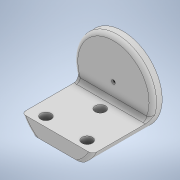
# Autodesk Inventor part: Adapter_Handgelenk
Saved by Autodesk Inventor 2022.2 (Build 262287010, 287A)
## iProperties
Created: 2024-02-12
Part Number: Adapter_Handgelenk
Material: Generisch
Document SubType Name: Modeling
Designer: ppovolni
Density: 1 g/cm^3
Appearance: Vorgabe
Author: ppovolni
Autodesk Inventor part; units mm, degrees
ref_plane "YZ Plane" through (0, 0, 0) normal (1, 0, 0) x (0, 1, 0)
ref_plane "XZ Plane" through (0, 0, 0) normal (0, 1, 0) x (-1, 0, 0)
ref_plane "XY Plane" through (0, 0, 0) normal (0, 0, 1) x (1, 0, 0)
sketch "Skizze1" plane through (0, 0, 0) normal (0, 0, 1) x (1, 0, 0)
  circle A0 centre (0, 0) radius 21
  dimension "d0" = 42
  constraints: 1 centre point, 1 coincident
  measures "d0" diameter of A0
extrude "Extrusion1" add sketch "Skizze1" along normal blind 5
sketch "Skizze2" plane through (0, 0, 0) normal (0, 0, -1) x (-1, 0, 0)
  circle A0 centre (0, 0) radius 2.35
  dimension "d3" = 4.7
  constraints: 1 centre point, 1 coincident
  measures "d3" diameter of A0
extrude "Extrusion2" cut sketch "Skizze2" against normal blind 4
sketch "Skizze3" plane through (0, 0, 4) normal (0, 0, -1) x (-1, 0, 0)
  circle A0 centre (0, 0) radius 1
  dimension "d6" = 2
  constraints: 1 centre point, 1 coincident
  measures "d6" diameter of A0
extrude "Extrusion3" cut sketch "Skizze3" against normal through all
sketch "Skizze4" plane through (0, 0, 5) normal (0, 0, 1) x (1, 0, 0)
  circle A0 centre (0, 0) radius 21 projected
  line L0 (-19, -8.9443) -> (19, -8.9443)
  dimension "d10" = 38
  constraints: 2 end point, 2 point on circle, 1 horizontal
  measures "d10" distance of L0.start L0.end
extrude "Extrusion4" add sketch "Skizze4" along normal blind 30 contours L0 A0 picked at (-5.5035, -10.2886)
fillet "Rundung1" radius 2 4 edges at (0, -8.9443, 5) (20.4939, -4.5826, 5) (-4.5826, 20.4939, 5) (0, -21, 35)
sketch "Skizze5" plane through (-17.6855, -8.9443, 7) normal (0, 1, 0) x (1, 0, 0)
  line L0 (15.3355, 7) -> (20.0355, 7) construction
  line L1 (-3.3145, 7) -> (38.6855, 7) construction
  line L2 (6.6855, 7) -> (28.6855, 7) construction
  line L3 (28.6855, 7) -> (28.6855, -23) construction
  line L4 (28.6855, -23) -> (6.6855, -23) construction
  line L5 (6.6855, -23) -> (6.6855, 7) construction
  line L6 (6.6855, -5) -> (28.6855, -5) construction
  circle A0 centre (17.6855, -5) radius 2.8
  circle A1 centre (28.6855, -23) radius 2.8
  circle A2 centre (6.6855, -23) radius 2.8
  line L7 (-1.3145, 0.1936) -> (-1.3145, -26) construction
  line L8 (36.6855, 0.1936) -> (36.6855, -26) construction
  line L9 (-1.3145, -26) -> (36.6855, -26) construction
  point P0 (17.6855, 7)
  point P1 (17.6855, -5)
  point P2 (17.6855, -26)
  dimension "d14" = 22
  dimension "d18" = 5.6
  dimension "d21" = 12
  dimension "d22" = 18
  dimension "d23" = 38
  constraints: 12 end point, 3 centre point, 3 coincident, 3 point on line, 2 equal radius, 2 horizontal, 2 midpoint, 2 parallel, 2 perpendicular, 1 vertical alignment
  measures "d14" distance of L3.end L4.end
  measures "d18" diameter of A0
  measures "d21" distance between parallel lines of L1 L6
  measures "d22" distance between parallel lines of L4 L6
  measures "d23" distance between parallel lines of L8 L7
extrude "Extrusion5" cut sketch "Skizze5" against normal through all
sketch "Skizze6" plane through (0, 0, 0) normal (0, 0, -1) x (-1, 0, 0)
  circle A0 centre (0, 0) radius 21 projected
  line L0 (-13.6015, -16) -> (13.6015, -16)
  dimension "d27" = 16
  constraints: 2 end point, 2 point on circle, 1 horizontal
  measures "d27" distance from line of L0 point (0, 0)
extrude "Extrusion6" cut sketch "Skizze6" against normal through all contours L0 A0 picked at (3.1683, -16.9086)
